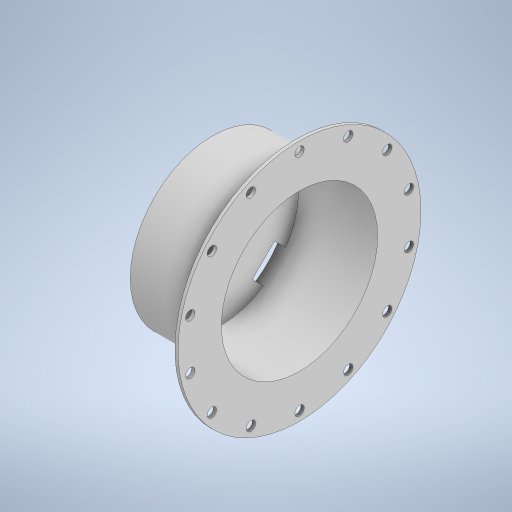
# Autodesk Inventor part: MotorCycDriveMount
Saved by Autodesk Inventor 2023 (Build 270158000, 158)
## iProperties
Created: 2023-02-23
Part Number: MotorCycDriveMount
Material: Generic
Document SubType Name: Sheet Metal
Designer: Charles Kelly
Density: 1 g/cm^3
Sheet Metal Rule: Default_mm
Appearance: Default
Author: Charles Kelly
Autodesk Inventor part; units mm, degrees
ref_plane "YZ Plane" through (0, 0, 0) normal (1, 0, 0) x (0, 1, 0)
ref_plane "XZ Plane" through (0, 0, 0) normal (0, 1, 0) x (-1, 0, 0)
ref_plane "XY Plane" through (0, 0, 0) normal (0, 0, 1) x (1, 0, 0)
sketch "Sketch1" plane through (0, 0, 0) normal (1, 0, 0) x (0, 1, 0)
  circle A0 centre (0, 0) radius 19
  circle A1 centre (0, -19) radius 1.75
  circle A2 centre (19, 0) radius 1.75
  circle A3 centre (0, 19) radius 1.75
  circle A4 centre (-19, 0) radius 1.75
  circle A5 centre (0, 0) radius 52.5
  circle A6 centre (0, 0) radius 40
  dimension "d0" = 38
  dimension "d1" = 3.5
  dimension "d4" = 360
  dimension "d6" = 105
  dimension "d7" = 80
  constraints: 6 centre point, 3 coincident, 1 vertical alignment, 11 other
  measures "d1" diameter of A1
  measures "d6" diameter of A5
  measures "d7" diameter of A6
extrude "Extrusion1" add sketch "Sketch1" along normal blind 5 contours A2 A0 A1 A4 A3 | A5 | A6
sketch "Sketch2" plane through (0, 0, 0) normal (-1, 0, 0) x (0, 0, 1)
  circle A0 centre (0, 0) radius 52.5
  circle A1 centre (0, 0) radius 49.875
  dimension "d10" = 105
  constraints: 2 centre point, 2 coincident
  measures "d10" diameter of A0
extrude "Extrusion2" add sketch "Sketch2" against normal blind 53.5
sketch "Sketch4" plane through (5, 0, 0) normal (1, 0, 0) x (0, 0, -1)
  circle A0 centre (0, 0) radius 15
  line L0 (0, 0) -> (7.0711, 7.0711)
  line L1 (0, 0) -> (10, 0) construction
  line L2 (7.0711, 7.0711) -> (41.6219, -27.4797)
  circle A1 centre (0, 0) radius 49.875 projected
  line L3 (0, 0) -> (-7.0711, -7.0711)
  line L4 (-7.0711, -7.0711) -> (27.4797, -41.6219)
  line L5 (41.6219, -27.4797) -> (34.5508, -20.4087)
  line L6 (34.5508, -20.4087) -> (20.4087, -34.5508)
  point P0 (0.8346, -14.9768)
  point P1 (14.9768, -0.8346)
  point P2 (-49.875, 0)
  point P3 (-49.875, 0)
  dimension "d27" = 30
  dimension "d28" = 10
  dimension "d29" = 45
  dimension "d30" = 10
  dimension "d34" = 10
  constraints: 14 end point, 3 perpendicular, 3 point on circle, 3 point on line, 1 centre point, 1 coincident, 1 equal length, 1 horizontal
  measures "d27" diameter of A0
  measures "d28" distance of L0.start L0.end
  measures "d29" angle of L1 L0
  measures "d30" distance of L3.start L3.end
  measures "d34" distance of L5.start L5.end
extrude "Extrusion4" cut sketch "Sketch4" against normal blind 10 contours A0 L2 L0 L3 L4 | L4 L3 L0 L2 A0 | L6 L2 A1 L4
sketch "Sketch6" plane through (53.5, 0, 0) normal (1, 0, 0) x (0, 0, -1)
  circle A0 centre (0, 0) radius 71.5
  circle A1 centre (0, 71.5) radius 3
  circle A2 centre (-55.901, 44.5795) radius 3
  circle A3 centre (-69.7073, -15.9102) radius 3
  circle A4 centre (-31.0227, -64.4193) radius 3
  circle A5 centre (31.0227, -64.4193) radius 3
  circle A6 centre (69.7073, -15.9102) radius 3
  circle A7 centre (55.901, 44.5795) radius 3
  circle A8 centre (0, 0) radius 15 projected
  circle A9 centre (0, 0) radius 77.5
  circle A10 centre (0, 0) radius 49.875
  circle A11 centre (-31.0227, 64.4193) radius 3
  circle A12 centre (-55.901, 44.5795) radius 3
  circle A13 centre (-69.7073, 15.9102) radius 3
  circle A14 centre (-69.7073, -15.9102) radius 3
  circle A15 centre (-55.901, -44.5795) radius 3
  circle A16 centre (-31.0227, -64.4193) radius 3
  circle A17 centre (0, -71.5) radius 3
  circle A18 centre (31.0227, -64.4193) radius 3
  circle A19 centre (55.901, -44.5795) radius 3
  circle A20 centre (69.7073, -15.9102) radius 3
  circle A21 centre (69.7073, 15.9102) radius 3
  circle A22 centre (55.901, 44.5795) radius 3
  circle A23 centre (31.0227, 64.4193) radius 3
  dimension "d35" = 143
  dimension "d36" = 6
  dimension "d39" = 360
  dimension "d41" = 155
  dimension "d46" = 360
  constraints: 22 centre point, 2 coincident, 1 vertical alignment, 46 other
  measures "d36" diameter of A1
  measures "d41" diameter of A9
extrude "Extrusion6" add sketch "Sketch6" along normal blind 2 contours A0 A6 A19 A5 A17 A4 A15 A3 A13 A2 A11 A1 A23 A7 A21 | A9
equation "\"BendRadius\" = Thickness"
equation "\"BendReliefWidth\" = Thickness"
equation "\"BendReliefDepth\" = 0.5 * Thickness"
equation "\"CornerReliefSize\" = 4 * Thickness"
equation "\"MinimumRemnant\" = 2 * Thickness"
equation "\"TransitionRadius\" = BendRadius"
equation "\"JacobiRadiusSize\" = BendRadius"
equation "\"GapSize\" = Thickness"
equation "\"Thickness\" = 0.5"
body "Solid1"
